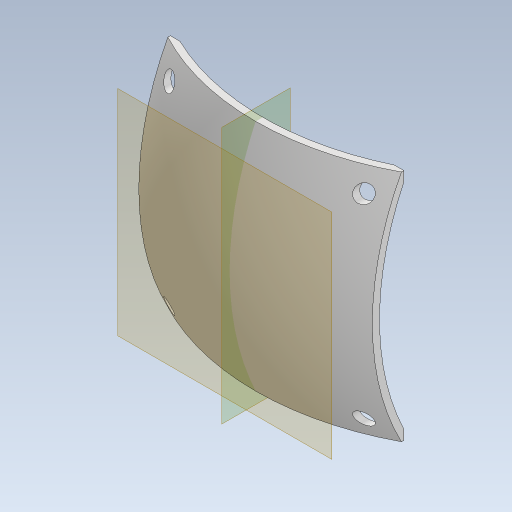
# Autodesk Inventor part: sling
Saved by Autodesk Inventor 2023 (Build 270158030, 158C)
## iProperties
Created: 2024-12-21
Part Number: sling
Material: Generic
Document SubType Name: Modeling
Designer: Imogen Heard
Density: 1 g/cm^3
Appearance: Default
Author: Imogen Heard
Autodesk Inventor part; units mm, degrees
ref_plane "YZ Plane" through (0, 0, 0) normal (1, 0, 0) x (0, 1, 0)
ref_plane "XZ Plane" through (0, 0, 0) normal (0, 1, 0) x (-1, 0, 0)
ref_plane "XY Plane" through (0, 0, 0) normal (0, 0, 1) x (1, 0, 0)
ref_plane "Work Plane1" through (0, 75, 0) normal (0, 0, 1) x (-1, 0, 0)
sketch "Sketch1" plane through (0, 75, 0) normal (0, 0, 1) x (-1, 0, 0)
  line L0 (-15, 15) -> (15, 15)
  line L1 (15, 15) -> (15, -15)
  line L2 (15, -15) -> (-15, -15)
  line L3 (-15, -15) -> (-15, 15)
  spline S0 degree 3 poles (-65.8465, 1.1295) (-66.0234, 1.0352) (-66.1848, 0.9117) (-66.4204, 0.6349) (-66.5034, 0.4929) (-66.5934, 0.2154) (-66.6116, 0.0884) (-66.6019, -0.1749) (-66.5715, -0.3066) (-66.4624, -0.5645) (-66.3819, -0.6861) (-66.1664, -0.9234) (-66.0248, -1.0312) (-65.6735, -1.2253) (-65.4553, -1.2976) (-64.959, -1.3795) (-64.675, -1.3719) (-64.1674, -1.2582) (-63.9381, -1.1635) (-63.5868, -0.9213) (-63.4527, -0.7919) (-63.2634, -0.5109) (-63.201, -0.3687) (-63.1464, -0.1021) (-63.1416, 0.0152) (-63.1732, 0.2716) (-63.2174, 0.4057) (-63.3546, 0.6619) (-63.4487, 0.7798) (-63.6944, 1.0081) (-63.8533, 1.1093) (-64.2408, 1.2828) (-64.4775, 1.3397) (-64.9073, 1.3715) (-65.1013, 1.3605) (-65.4835, 1.2866) (-65.6727, 1.2221) (-65.8465, 1.1295) knots 0 0 0 0 0.060136 0.060136 0.109397 0.109397 0.148117 0.148117 0.188879 0.188879 0.232535 0.232535 0.285353 0.285353 0.353015 0.353015 0.435935 0.435935 0.508779 0.508779 0.564183 0.564183 0.610882 0.610882 0.646334 0.646334 0.688872 0.688872 0.733954 0.733954 0.789815 0.789815 0.861387 0.861387 0.918865 0.918865 0.977951 0.977951 0.977951 0.977951 projected
  line L4 (50, 27.5) -> (-50, 27.5) projected
  line L5 (-50, -27.5) -> (50, -27.5) projected
  point P0 (0, 75)
  point P1 (-65.8465, 1.1295)
  dimension "d0" = 30
  dimension "d1" = 30
  dimension "d2" = 15
  dimension "d3" = 12.5
  dimension "d4" = 12.5
  constraints: 8 end point, 2 parallel, 1 horizontal, 1 perpendicular
  measures "d0" distance between parallel lines of L1 L3
  measures "d1" distance between parallel lines of L2 L0
  measures "d2" distance from line of L3 point (0, 75)
  measures "d3" distance between parallel lines of L0 L4
  measures "d4" distance between parallel lines of L5 L2
extrude "Extrusion1" add sketch "Sketch1" against normal blind 8 contours L0 L1 L2 L3
ref_plane "Work Plane2" through (0, 60, 0) normal (-1, 0, 0) x (0, 0, 1)
sketch "Sketch2" plane through (0, 60, 0) normal (-1, 0, 0) x (0, 0, 1)
  line L0 (0, 30) -> (0, 0) projected
  line L1 (0, 30) -> (-8, 30) projected
  line L2 (-8, 0) -> (-8, 30) projected
  line L3 (0, 0) -> (-8, 0) projected
  line L4 (-15.437, 15) -> (9.9461, 15)
  line L5 (0, 0) -> (-8, 0) projected
  line L6 (0, 0) -> (-8, 0) projected
  line L7 (0, 30) -> (-8, 30) projected
  line L8 (-6, 0) -> (-8, 0)
  line L9 (-6, 30) -> (-8, 30)
  line L10 (0, 0) -> (-8, 0)
  line L11 (-8, 30) -> (0, 30)
  line L12 (0, 0) -> (0, 30) projected
  line L13 (0, 0) -> (-8, 0)
  line L14 (-8, 0) -> (-8, -11)
  line L15 (-8, -11) -> (0, -11)
  line L16 (0, -11) -> (0, 0)
  line L17 (-8, 30) -> (0, 30)
  line L18 (0, 30) -> (0, 41)
  line L19 (0, 41) -> (-8, 41)
  line L20 (-8, 41) -> (-8, 30)
  arc A0 (-12, -11) -> (-12, 41) centre (-35.9838, 15) ccw
  arc A1 (-13, -11) -> (-13, 41) centre (-36.631, 15) ccw
  point P0 (0, -60)
  point P1 (-4, 0)
  point P2 (-8, 15)
  point P3 (0, 15)
  point P4 (-6, 0)
  point P5 (-8, -5.3639)
  point P6 (-1.4966, 15)
  point P7 (-0.6112, 15)
  point P8 (-8, -6.6363)
  dimension "d9" = 15
  dimension "d19" = 15
  dimension "d20" = 11
  dimension "d21" = 11
  dimension "d22" = 4
  dimension "d23" = 1
  constraints: 26 end point, 5 horizontal, 5 horizontal alignment, 5 vertical alignment, 4 coincident, 4 parallel, 4 point on circle, 3 point on line, 2 centre point, 2 collinear, 2 perpendicular, 1 midpoint
  measures "d9" distance between parallel lines of L4 L1
  measures "d19" distance between parallel lines of L3 L4
  measures "d20" distance between parallel lines of L15 L3
  measures "d21" distance between parallel lines of L1 L19
  measures "d22" horizontal distance of A0.start L2.start
  measures "d23" distance of A1.start A0.start
revolve "Revolution1" cut sketch "Sketch2" angle 360 about axis through (0, 75, -15.437) along (0, 0, 1) contours L0 L3 A0 L4 | L16 L15 L14 A0 L3 | A1 L3 L2 L4 | A1 L14 L3
sketch "Sketch3" plane through (0, 75, -8) normal (0, 0, -1) x (-1, 0, 0)
  circle A0 centre (-12.5, -12.5) radius 1
  line L0 (-15, -13.7728) -> (-15, -15) projected
  line L1 (-15, -15) -> (-13.7728, -15) projected
  circle A1 centre (12.5, -12.5) radius 1
  circle A2 centre (-12.5, 12.5) radius 1
  circle A3 centre (12.5, 12.5) radius 1
  line L2 (15, 13.7728) -> (15, 15) projected
  line L3 (15, 15) -> (13.7728, 15) projected
  point P0 (0, -75)
  dimension "d24" = 2
  dimension "d25" = 2.5
  dimension "d26" = 2.5
  dimension "d27" = 2.5
  dimension "d28" = 2.5
  constraints: 4 centre point, 3 equal radius, 2 horizontal alignment, 2 vertical alignment
  measures "d24" diameter of A0
  measures "d25" distance from line of L0 A0.centre
  measures "d26" distance from line of L1 A0.centre
  measures "d27" distance from line of L2 A3.centre
  measures "d28" distance from line of L3 A3.centre
extrude "Extrusion2" cut sketch "Sketch3" against normal through all
equation "\"d1\" = d0"
equation "\"d25\" = d28"
equation "\"d26\" = d27"
